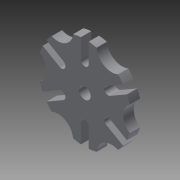
# Autodesk Inventor part: Geneva Driven
Saved by Autodesk Inventor 2018 (Build 220112000, 112)
## iProperties
Created: 2018-01-19
Part Number: Geneva Driven
Material: Generic
Document SubType Name: Modeling
Designer: Rus
Density: 1 g/cm^3
Appearance: Default
Author: Rus
Autodesk Inventor part; units mm, degrees
ref_plane "YZ Plane" through (0, 0, 0) normal (1, 0, 0) x (0, 1, 0)
ref_plane "XZ Plane" through (0, 0, 0) normal (0, 1, 0) x (-1, 0, 0)
ref_plane "XY Plane" through (0, 0, 0) normal (0, 0, 1) x (1, 0, 0)
sketch "Sketch2" plane through (0, 0, 0) normal (0, 0, 1) x (1, 0, 0)
  line L0 (0, 0) -> (87.9881, 0) construction
  line L1 (0, 0) -> (65.9905, 38.1011) construction
  line L2 (65.9905, 38.1011) -> (87.9881, 0) construction
  circle A0 centre (0, 0) radius 76.2 construction
  line L3 (62.5859, 43.4678) -> (34.9256, 27.4975)
  line L4 (68.9361, 32.4694) -> (41.2758, 16.4991)
  arc A1 (34.9256, 27.4975) -> (41.2758, 16.4991) centre (38.1007, 21.9983) ccw
  arc A2 (73.4536, 20.2735) -> (73.4536, -20.2735) centre (87.9881, 0) ccw
  arc A3 (73.4536, 20.2735) -> (68.9361, 32.4694) centre (0, 0) ccw
  line L5 (62.5873, -43.4657) -> (34.9265, -27.4963)
  arc A4 (41.2764, -16.4977) -> (34.9265, -27.4963) centre (38.1014, -21.997) ccw
  line L6 (68.9371, -32.4671) -> (41.2764, -16.4977)
  arc A5 (54.2842, -53.4759) -> (62.5873, -43.4657) centre (0, 0) ccw
  arc A6 (54.2842, -53.4759) -> (19.1694, -73.7494) centre (43.9941, -76.2) ccw
  line L7 (-6.3487, -75.9351) -> (-6.3493, -43.9954)
  arc A7 (6.3507, -43.9952) -> (-6.3493, -43.9954) centre (0.0007, -43.9953) ccw
  line L8 (6.3513, -75.9348) -> (6.3507, -43.9952)
  arc A8 (-19.1694, -73.7494) -> (-6.3487, -75.9351) centre (0, 0) ccw
  arc A9 (-19.1694, -73.7494) -> (-54.2842, -53.4759) centre (-43.9941, -76.2) ccw
  line L9 (-68.9361, -32.4694) -> (-41.2758, -16.4991)
  arc A10 (-34.9256, -27.4975) -> (-41.2758, -16.4991) centre (-38.1007, -21.9983) ccw
  line L10 (-62.5859, -43.4678) -> (-34.9256, -27.4975)
  arc A11 (-73.4536, -20.2735) -> (-68.9361, -32.4694) centre (0, 0) ccw
  arc A12 (-73.4536, -20.2735) -> (-73.4536, 20.2735) centre (-87.9881, 0) ccw
  line L11 (-62.5873, 43.4657) -> (-34.9265, 27.4963)
  arc A13 (-41.2764, 16.4977) -> (-34.9265, 27.4963) centre (-38.1014, 21.997) ccw
  line L12 (-68.9371, 32.4671) -> (-41.2764, 16.4977)
  arc A14 (-54.2842, 53.4759) -> (-62.5873, 43.4657) centre (0, 0) ccw
  arc A15 (-54.2842, 53.4759) -> (-19.1694, 73.7494) centre (-43.9941, 76.2) ccw
  line L13 (6.3487, 75.9351) -> (6.3493, 43.9954)
  arc A16 (-6.3507, 43.9952) -> (6.3493, 43.9954) centre (-0.0007, 43.9953) ccw
  line L14 (-6.3513, 75.9348) -> (-6.3507, 43.9952)
  arc A17 (19.1694, 73.7494) -> (6.3487, 75.9351) centre (0, 0) ccw
  arc A18 (19.1694, 73.7494) -> (54.2842, 53.4759) centre (43.9941, 76.2) ccw
  arc A19 (62.5859, 43.4678) -> (54.2842, 53.4759) centre (0, 0) ccw
  arc A20 (-6.3513, 75.9348) -> (-19.1694, 73.7494) centre (0, 0) ccw
  arc A21 (-68.9371, 32.4671) -> (-73.4536, 20.2735) centre (0, 0) ccw
  arc A22 (-62.5859, -43.4678) -> (-54.2842, -53.4759) centre (0, 0) ccw
  arc A23 (6.3513, -75.9348) -> (19.1694, -73.7494) centre (0, 0) ccw
  arc A24 (68.9371, -32.4671) -> (73.4536, -20.2735) centre (0, 0) ccw
  dimension "d6" = 87.9881
  dimension "d7" = 43.9953
  dimension "d8" = 76.2
  dimension "d9" = 12.7
  dimension "d10" = 32.2047
  dimension "d12" = 24.9453
  dimension "d15" = 360
  constraints: 53 point on circle, 30 end point, 25 centre point, 8 coincident, 2 parallel, 2 tangent, 1 concentric, 1 horizontal, 1 point on line, 85 other
  measures "d6" distance of L0.start L0.end
  measures "d7" distance of L1.end L0.end
  measures "d8" distance of L0.start L1.end
  measures "d9" distance between parallel lines of L3 L4
  measures "d10" distance of L1.end A1.centre
  measures "d12" radius of A2
extrude "Extrusion1" add sketch "Sketch2" along normal blind 16.9333
sketch "Sketch3" plane through (0, 0, 16.9333) normal (0, 0, 1) x (1, 0, 0)
  circle A0 centre (0, 0) radius 9.525
  dimension "d19" = 19.05
  constraints: 1 centre point, 1 coincident
  measures "d19" diameter of A0
extrude "Extrusion2" cut sketch "Sketch3" against normal through all
body "Solid1"
